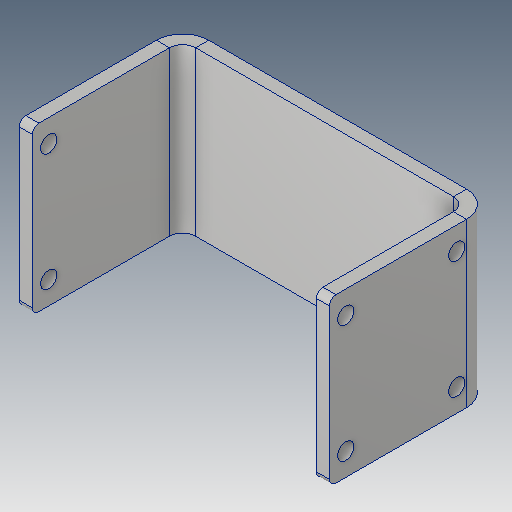
# Autodesk Inventor part: coluna-apoio
Saved by Autodesk Inventor 2017 (Build 210142000, 142)
## iProperties
Created: 2018-06-21
Part Number: coluna-apoio
Material: Aluminum 6061
Document SubType Name: Sheet Metal
Designer: Luiz Gustavo
Density: 2.7 g/cm^3
Sheet Metal Rule: Default_mm
Appearance: Aluminum - Flat
Flat Pattern Width: 5 cm
Flat Pattern Length: 18.1096 cm
Flat Pattern Area: 90.5478 cm^2
Sheet Metal Width: 50,000 mm
Sheet Metal Length: 181,096 mm
Sheet Metal Area: 9054,779 mm^2
Mass: 96.8893 g
Surface Area: 201.605 cm^2
Volume: 35.8849 cm^3
Author: Luiz Gustavo
Autodesk Inventor part; units mm, degrees
ref_plane "YZ Plane" through (0, 0, 0) normal (1, 0, 0) x (0, 1, 0)
ref_plane "XZ Plane" through (0, 0, 0) normal (0, 1, 0) x (-1, 0, 0)
ref_plane "XY Plane" through (0, 0, 0) normal (0, 0, 1) x (1, 0, 0)
sketch "Sketch1" plane through (0, 0, 0) normal (0, 0, 1) x (1, 0, 0)
  line L0 (-47.5, 25) -> (47.5, 25)
  line L1 (47.5, 25) -> (47.5, -25)
  line L2 (47.5, -25) -> (-47.5, -25)
  line L3 (-47.5, -25) -> (-47.5, 25)
  line L4 (-47.5, 25) -> (47.5, -25) construction
  line L5 (47.5, 25) -> (-47.5, -25) construction
  point P0 (0, 0)
  dimension "d0" = 50
  dimension "d20" = 95
  measures "d0" distance of L2.end L0.start
  measures "d20" distance of L0.start L0.end
extrude "Plate1" add sketch "Sketch1" along normal blind 4
sketch "Sketch2" plane through (-43.5, -25, 0) normal (-1, 0, 0) x (0, -1, 0)
  line L0 (-50, 0) -> (0, 0)
  line L1 (0, 0) -> (0, 50)
  line L2 (0, 50) -> (-50, 50)
  line L3 (-50, 50) -> (-50, 0)
  constraints: 6 end point, 1 horizontal, 1 perpendicular, 1 vertical
edge flange "Flange1" height 50 angle 90 thickness 4 bend radius 4 thickness toward (-1, 0, 0) relief tear relief width 4 relief depth 2 corner gap 4 corner form 0 edges at (-47.5, 0, 4) (47.5, 0, 4) wall of the first edge with corners at (-43.5, 25, 0) (-43.5, -25, 0) (-43.5, -25, 50) (-43.5, 25, 50)
bend "Bend1"
corner "Corner1"
sketch "Sketch3" plane through (0, 0, 0) normal (1, 0, 0) x (0, 1, 0)
  line L0 (25, 8) -> (25, 50) projected
  line L1 (25, 50) -> (-25, 50) projected
  line L2 (-25, 50) -> (-25, 8) projected
  line L3 (-18, 11) -> (18, 11) construction
  line L4 (18, 11) -> (18, 45) construction
  line L5 (18, 45) -> (-18, 45) construction
  line L6 (-18, 45) -> (-18, 11) construction
  line L7 (-18, 11) -> (18, 45) construction
  line L8 (18, 11) -> (-18, 45) construction
  circle A0 centre (18, 45) radius 2.5
  circle A1 centre (-18, 45) radius 2.5
  circle A2 centre (-18, 11) radius 2.5
  circle A3 centre (18, 11) radius 2.5
  point P0 (0, 0)
  point P1 (0, 28)
  dimension "d12" = 5
  dimension "d13" = 7
  dimension "d14" = 7
  dimension "d15" = 34
  dimension "d16" = 5
  constraints: 12 end point, 4 centre point, 4 coincident, 3 equal radius, 2 midpoint, 2 parallel, 1 horizontal, 1 perpendicular
  measures "d12" distance between parallel lines of L5 L1
  measures "d13" distance between parallel lines of L4 L0
  measures "d14" distance between parallel lines of L2 L6
  measures "d15" distance between parallel lines of L3 L5
  measures "d16" diameter of A0
extrude "Extrusion1" cut sketch "Sketch3" along normal through all both and the other way through all contours A0 | A1
fillet "Fillet1" radius 2 4 edges at (-45.5, 25, 50) (-45.5, -25, 50) (45.5, 25, 50) (45.5, -25, 50)
extrude "Extrusion2" cut sketch "Sketch3" along normal through all contours A2 | A3
equation "\"d14\" = d13"
equation "\"d2\" = BendReliefWidth"
equation "\"d3\" = BendReliefDepth"
equation "\"d4\" = MinimumRemnant"
equation "\"d5\" = BendRadius"
equation "\"d8\" = BendRadius"
equation "\"d9\" = CornerReliefSize"
equation "\"d10\" = GapSize"
equation "\"d11\" = JacobiRadiusSize"
equation "\"BendRadius\" = Thickness"
equation "\"BendReliefWidth\" = Thickness"
equation "\"BendReliefDepth\" = 0.5 * Thickness"
equation "\"CornerReliefSize\" = 4 * Thickness"
equation "\"MinimumRemnant\" = 2 * Thickness"
equation "\"TransitionRadius\" = BendRadius"
equation "\"JacobiRadiusSize\" = BendRadius"
equation "\"GapSize\" = Thickness"
equation "\"d1\" = BendRadius"
equation "\"Thickness\" = 4"
body "Solid1"
